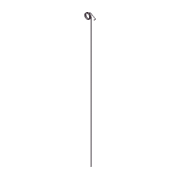
# Autodesk Inventor part: antenna_rx_deploy
Saved by Autodesk Inventor 2014 SP1 (Build 180222100, 222)
## iProperties
Created: 2012-11-10
Document SubType Name: Modeling
Designer: Robert Davis
Density: 8.36 g/cm^3
Material: BeCu
Mass: 0.436871 g
Surface Area: 4.18903 cm^2
Volume: 0.0522572 cm^3
Description: TORSION SPRING ANTENNA
Part Number: antenna_rx_deploy
Appearance: Copper - Satin
Author: Robert Davis
Autodesk Inventor part; units mm, degrees
ref_plane "YZ Plane" through (0, 0, 0) normal (1, 0, 0) x (0, 1, 0)
ref_plane "XZ Plane" through (0, 0, 0) normal (0, 1, 0) x (-1, 0, 0)
sketch "Sketch1" plane through (0, 0, 0) normal (0, 0, 1) x (1, 0, 0)
  circle A0 centre (0, 0) radius 0.25
  line L0 (-3.175, 0) -> (-3.175, 4.9243)
  dimension "d0" = 0.5
  dimension "d1" = 6.35
  constraints: 2 end point, 1 centre point, 1 vertical
  measures "d0" diameter of A0
  measures "d1" diameter of point (0, 0) L0
coil "Coil1" sketch "Sketch1" operation add axis through (-3.175, 0, 0) along (0, 1, 0) pitch 0.51 turns 4 hand right
ref_plane "Work Plane2" through (0, 0, 0) normal (0, -0.0393, 0.9992) x (1, 0, 0)
ref_plane "Work Plane3" through (0, 0, 0) normal (0, -0.9992, -0.0393) x (1, 0, 0)
sketch "Sketch2" plane through (0, 0, 0) normal (0, -0.0393, 0.9992) x (1, 0, 0)
  circle A0 centre (0, 0) radius 0.25
  circle A1 centre (0, 0) radius 0.25
  point P0 (0.25, 0)
  dimension "d10" = 0.5
  constraints: 1 centre point, 1 horizontal alignment, 1 other
  measures "d10" diameter of A1
sketch3d "3D Sketch2"
  line L0 (0, 0, 0) -> (0, 0, 5.2679)
  arc A0 (0, 0, 5.2679) -> (1.5, 0, 6.134) centre (1, 0, 5.2679) ccw
  line L1 (1.5, 0, 6.134) -> (7.2746, 0, 2.8)
  arc A1 (7.2746, 0, 2.8) -> (7.7942, -0.6, 2.5) centre (7.2746, -0.6, 2.8) ccw
  line L2 (7.7942, -0.6, 2.5) -> (7.7942, -2.0306, 2.5)
  dimension "d20" = 7
  dimension "d37" = 0.6
  dimension "d40" = 9
  dimension "d41" = 60
  dimension "d36" = 1
  constraints: 2 vertical
sweep "Sweep1" add profiles "Sketch2" path "3D Sketch2"
sketch "Sketch6" plane through (0, 2.04, 0) normal (0, 0, -1) x (-1, 0, 0)
  circle A0 centre (0, 0) radius 0.25 projected
  circle A1 centre (0, 0) radius 0.25
  point P0 (-0.25, 0)
  point P1 (0, -2.04)
  constraints: 1 centre point, 1 horizontal alignment
extrude "Extrusion1" add sketch "Sketch6" along normal blind 165
body "Solid1"
